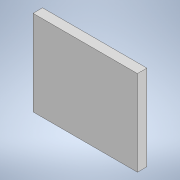
# Autodesk Inventor part: 應變規
Saved by Autodesk Inventor 2022 (Build 260153000, 153)
## iProperties
Created: 2023-03-14
Part Number: 應變規
Material: 一般
Document SubType Name: Modeling
Designer: User
Mass: 0.792 g
Surface Area: 9.52 cm^2
Volume: 0.792 cm^3
Density: 1 g/cm^3
Appearance: 預設
Author: User
Autodesk Inventor part; units mm, degrees
ref_plane "YZ Plane" through (0, 0, 0) normal (1, 0, 0) x (0, 1, 0)
ref_plane "XZ Plane" through (0, 0, 0) normal (0, 1, 0) x (-1, 0, 0)
ref_plane "XY Plane" through (0, 0, 0) normal (0, 0, 1) x (1, 0, 0)
sketch "草圖1" plane through (0, 0, 0) normal (0, 0, 1) x (1, 0, 0)
  line L0 (-11, 9) -> (11, 9)
  line L1 (11, 9) -> (11, -9)
  line L2 (11, -9) -> (-11, -9)
  line L3 (-11, -9) -> (-11, 9)
  line L4 (-15.4, 0) -> (15.4, 0) construction
  line L5 (0, -12.6) -> (0, 12.6) construction
  point P0 (0, 0)
  point P1 (0, 9)
  point P2 (11, 0)
  dimension "d0" = 18
  dimension "d1" = 22
  constraints: 8 end point, 2 midpoint, 2 parallel, 2 point on line, 1 horizontal, 1 perpendicular
  measures "d0" distance of L0.end L1.end
  measures "d1" distance of L0.start L0.end
extrude "擠出1" add sketch "草圖1" along normal blind 2
